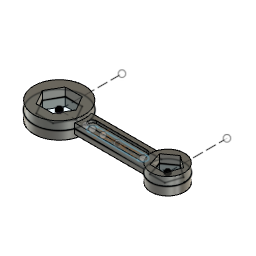
exercise 2 v1 (Autodesk Fusion 360 design; units mm, degrees)
Autodesk Fusion 360 part; units mm, degrees
sketch "Sketch1" plane through (0, 0, 0) normal (0, 0, 1) x (1, 0, 0) in component "exercise 2"
  circle A0 centre (0, 0) radius 30
  line L0 (0, 0) -> (129, 0) construction
  circle A1 centre (129, 0) radius 20
  line L1 (0, 0) -> (0, 74.6683) construction
  line L2 (129, 0) -> (129, 70.5762) construction
  line L3 (-20, 0) -> (-10, -17.3205)
  line L4 (-10, -17.3205) -> (10, -17.3205)
  line L5 (10, -17.3205) -> (20, 0)
  line L6 (20, 0) -> (10, 17.3205)
  line L7 (10, 17.3205) -> (-10, 17.3205)
  line L8 (-10, 17.3205) -> (-20, 0)
  line L9 (129, 15) -> (114.7342, 4.6353)
  line L10 (114.7342, 4.6353) -> (120.1832, -12.1353)
  line L11 (120.1832, -12.1353) -> (137.8168, -12.1353)
  line L12 (137.8168, -12.1353) -> (143.2658, 4.6353)
  line L13 (143.2658, 4.6353) -> (129, 15)
  line L14 (30, 0) -> (31.5826, 0)
  line L15 (28.2843, 10) -> (111.6795, 10)
  line L16 (28.2843, -10) -> (111.6795, -10)
  line L17 (50, 10) -> (50, -10) construction
  line L18 (50, 0) -> (52, 0)
  line L19 (99.5, -5) -> (39.5, -5)
  line L20 (39.5, 5) -> (99.5, 5)
  line L21 (99.5, -5) -> (39.5, 5) construction
  line L22 (39.5, -5) -> (99.5, 5) construction
  arc A2 (41.1216, 4.7297) -> (41.1216, -4.7297) centre (39.5, 0) ccw
  arc A3 (97.8784, -4.7297) -> (97.8784, 4.7297) centre (99.5, 0) ccw
  point P0 (129, 0)
  point P1 (69.5, 0)
  dimension "d1" = 60
  dimension "d2" = 40
  dimension "d3" = 129
  dimension "d4" = 20
  dimension "d5" = 15
  dimension "d6" = 20
  dimension "d9" = 60
  constraint coincident A0.centre L0.start
  constraint horizontal L0
  constraint coincident P0 L0.end
  constraint vertical L1
  constraint vertical L2
  constraint horizontal L7
  constraint coincident L2 L9.start
  constraint coincident A0 L14.start
  constraint coincident A0.centre L14
  constraint horizontal L14
  constraint coincident A1 L16.end
  constraint horizontal L16
  constraint horizontal L15
  constraint coincident L15 L17.start
  constraint perpendicular L15 L17
  constraint coincident L16 L17.end
  constraint midpoint L17 L18.start
  constraint perpendicular L17 L18
  constraint collinear L0 L18
  constraint coincident A0 L15.start
  constraint coincident A0 L16.start
  constraint coincident A1 L15.end
  constraint horizontal L19
  constraint parallel L19 L20
  constraint coincident L21 P1
  constraint coincident L22 P1
  constraint coincident L20.start A2
  constraint tangent L20 A2
  constraint coincident L19.end A2
  constraint coincident L20.end A3
  constraint tangent L20 A3
  constraint coincident L19.start A3
  constraint coincident L21 A2.start
  constraint coincident L22 A2.end
  constraint coincident L22 A3.end
  constraint coincident L21 A3.start
  measures "d1" diameter of A0
  measures "d2" diameter of A1
  measures "d3" distance of A0.centre P0
  measures "d4" distance of L3.start A0.centre
  measures "d5" distance of L9.start P0
  measures "d6" distance of L15 L16
  measures "d9" distance of L20.start L20.end
extrude "Extrude1" add sketch "Sketch1" along normal mid plane 20 contours A0 | A1 makes body 1 at (18.836, -10.4559, 10) makes body 2 at (148.9006, -1.9914, -3.3333) in component "exercise 2"
extrude "Extrude2" add sketch "Sketch1" along normal mid plane 12 contours A0 A1 L15 L16 bodies 1 2 in component "exercise 2"
extrude "Extrude3" add sketch "Sketch1" along normal mid plane 6 contours L19 L20 A2 A3 bodies 1 in component "exercise 2"
component "exercise 2" placed x (1, 0, 0) y (0, 1, 0) z (0, 0, 1) at (0, 0, 0)
